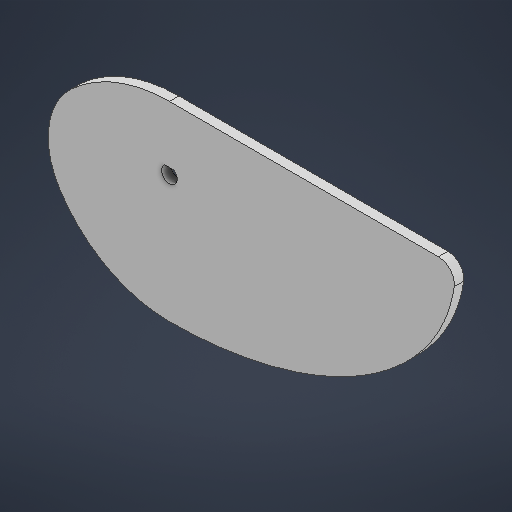
# Autodesk Inventor part: cam3
Saved by Autodesk Inventor 2027 (Build 310192000, 192)
## iProperties
Created: 2026-05-11
Part Number: cam3
Material: Generic
Document SubType Name: Modeling
Designer: alexy
Density: 1 g/cm^3
Appearance: Default
Author: alexy
Autodesk Inventor part; units mm, degrees
ref_plane "YZ Plane" through (0, 0, 0) normal (1, 0, 0) x (0, 1, 0)
ref_plane "XZ Plane" through (0, 0, 0) normal (0, 1, 0) x (-1, 0, 0)
ref_plane "XY Plane" through (0, 0, 0) normal (0, 0, 1) x (1, 0, 0)
sketch "Sketch1" plane through (0, 0, 0) normal (0, 0, 1) x (1, 0, 0)
  ellipse E0 centre (0, 0) end of major axis (90, 0) minor radius 60 (0, -60) -> (90, 0) ccw
  line L0 (0, 0) -> (90, 0)
  line L1 (0, -60) -> (0, 0)
  arc A0 (-34.5293, -41.1535) -> (0, -60) centre (0, -18.9457) ccw
  arc A1 (-30.6814, -11.8648) -> (-34.5293, -41.1535) centre (-15.2956, -28.7832) ccw
  arc A2 (0, 0) -> (-30.6814, -11.8648) centre (0, -45.6024) ccw
  point P0 (-30.1245, -11.3745)
  dimension "d0" = 90
  dimension "d1" = 60
  constraints: 7 point on circle, 4 end point, 3 centre point, 3 tangent, 1 coincident, 1 horizontal, 1 vertical, 5 other
  measures "d0" distance of point (0, 0) L0.end
  measures "d1" distance of L0.start L1.start
extrude "Extrusion1" add sketch "Sketch1" along normal blind 3
fillet "Fillet1" radius 5 1 edges at (90, 0, 1.5)
sketch "Sketch2" plane through (0, 0, 3) normal (0, 0, 1) x (1, 0, 0)
  arc A0 (-1.5, -18) -> (1.5, -18) centre (0, -20) ccw
  line L0 (-1.5, -18) -> (1.5, -18)
  point P0 (0, 0)
  dimension "d5" = 5
  dimension "d6" = 20
  dimension "d7" = 2
  constraints: 2 end point, 2 point on circle, 1 centre point, 1 horizontal, 1 vertical alignment
  measures "d5" diameter of A0
  measures "d6" distance of point (0, 0) A0.centre
  measures "d7" distance from line of L0 A0.centre
extrude "Extrusion2" cut sketch "Sketch2" against normal blind 3
body "Solid1"
